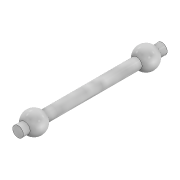
# Autodesk Inventor part: Delts Robot Arm Joint Rod
Saved by Autodesk Inventor 2020 (Build 240168000, 168)
## iProperties
Created: 2021-03-06
Part Number: Delts Robot Arm Joint Rod
Material: Generic
Document SubType Name: Modeling
Designer: Coy
Density: 1 g/cm^3
Appearance: Flat - Polished Gray
Author: Coy
Autodesk Inventor part; units mm, degrees
ref_plane "YZ Plane" through (0, 0, 0) normal (1, 0, 0) x (0, 1, 0)
ref_plane "XZ Plane" through (0, 0, 0) normal (0, 1, 0) x (-1, 0, 0)
ref_plane "XY Plane" through (0, 0, 0) normal (0, 0, 1) x (1, 0, 0)
sketch "Sketch1" plane through (0, 0, 0) normal (0, 1, 0) x (-1, 0, 0)
  line L0 (0, 0) -> (0, 27) construction
  line L1 (0, 0) -> (0, 1.2679)
  line L2 (0, 4.7321) -> (0, 22.2679)
  line L3 (0, 27) -> (0, 25.7321)
  line L4 (-1, 30.1625) -> (-1, -2.7373)
  line L5 (0, 27) -> (-1, 27)
  line L6 (0, 0) -> (-1, 0)
  line L7 (0, 26) -> (0, 22) construction
  line L8 (0, 24) -> (-1, 24) construction
  circle A0 centre (-1, 24) radius 2
  line L9 (0, 5) -> (0, 1) construction
  line L10 (0, 3) -> (-1, 3) construction
  circle A1 centre (-1, 3) radius 2
  dimension "d0" = 27
  dimension "d8" = 1
  dimension "d9" = 4
  dimension "d10" = 4
  constraints: 22 end point, 11 point on line, 4 perpendicular, 4 point on circle, 2 centre point, 2 coincident, 2 collinear, 2 midpoint, 2 vertical
  measures "d0" distance of L0.start L0.end
  measures "d8" distance between parallel lines of L0 L4
  measures "d9" diameter of A0
  measures "d10" diameter of A1
revolve "Revolution1" add sketch "Sketch1" angle 360 about axis through (1, 0, 30.1625) along (0, 0, -1) picked at (-0.5539, 3.4954) picked at (-0.772, 24.6265) contours L6 L4 A1 L1 | A1 L4 | A1 L4 A0 L2 | A0 L4 | L4 L5 L3 A0
body "Solid1"
